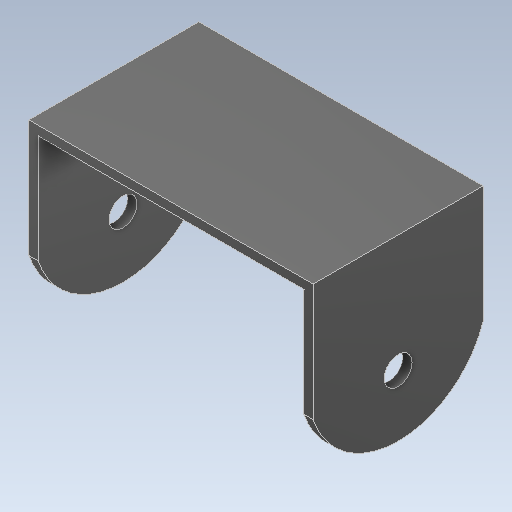
# Autodesk Inventor part: atassolar
Saved by Autodesk Inventor 2025.1 (Build 291241000, 241)
## iProperties
Created: 2024-11-08
Part Number: atassolar
Material: Aluminum 6061
Document SubType Name: Modeling
Designer: ramad
Density: 2.7 g/cm^3
Appearance: Aluminum - Flat
Author: ramad
Autodesk Inventor part; units mm, degrees
ref_plane "YZ Plane" through (0, 0, 0) normal (1, 0, 0) x (0, 1, 0)
ref_plane "XZ Plane" through (0, 0, 0) normal (0, 1, 0) x (-1, 0, 0)
ref_plane "XY Plane" through (0, 0, 0) normal (0, 0, 1) x (1, 0, 0)
sketch "Sketch1" plane through (0, 0, 0) normal (0, 1, 0) x (-1, 0, 0)
  line L0 (-43, 27.5) -> (43, 27.5)
  line L1 (43, 27.5) -> (43, -27.5)
  line L2 (43, -27.5) -> (-43, -27.5)
  line L3 (-43, -27.5) -> (-43, 27.5)
  line L4 (-43, 27.5) -> (43, -27.5) construction
  line L5 (43, 27.5) -> (-43, -27.5) construction
  line L6 (43, -27.5) -> (46, -27.5)
  line L7 (46, -27.5) -> (46, 27.5)
  line L8 (46, 27.5) -> (43, 27.5)
  line L9 (43, 27.5) -> (43, -27.5)
  line L10 (-43, -27.5) -> (-46, -27.5)
  line L11 (-46, -27.5) -> (-46, 27.5)
  line L12 (-46, 27.5) -> (-43, 27.5)
  line L13 (-43, 27.5) -> (-43, -27.5)
  point P0 (0, 0)
  dimension "d0" = 86
  dimension "d1" = 55
  dimension "d2" = 3
  dimension "d3" = 55
  dimension "d4" = 3
  constraints: 28 end point, 6 parallel, 3 horizontal, 3 perpendicular, 2 midpoint, 1 point on line
  measures "d0" distance of L1.end L2.end
  measures "d1" distance of L0.end L1.end
  measures "d2" distance of L8.end L7.end
  measures "d3" distance of L7.end L6.end
  measures "d4" distance of L11.end L12.end
extrude "Extrusion1" add sketch "Sketch1" along normal blind 3 contours L0 L1 L2 L3
extrude "Extrusion2" add sketch "Sketch1" along normal blind 3 contours L3 L10 L11 L12 | L8 L7 L6 L1
extrude "Extrusion3" add sketch "Sketch1" against normal blind 35 contours L3 L10 L11 L12 | L8 L7 L6 L1
sketch "Sketch2" plane through (46, 3, 27.5) normal (1, 0, 0) x (0, 0, -1)
  line L0 (0, -3) -> (0, -38) projected
  line L1 (0, -38) -> (55, -38) projected
  arc A0 (0, -38) -> (55, -38) centre (27.5, -28.794) ccw
  point P0 (27.5, -3)
  dimension "d11" = 29
  constraints: 2 point on circle, 1 centre point
  measures "d11" radius of A0
extrude "Extrusion4" add sketch "Sketch2" against normal up to surface (3 mm away)
mirror "Mirror1" about plane through (0, 0, 0) normal (1, 0, 0) of "Extrusion4"
sketch "Sketch3" plane through (-46, 3, -27.5) normal (-1, 0, 0) x (0, 0, 1)
  circle A0 centre (27.5, -38) radius 4.5
  point P0 (27.5, -3)
  point P1 (0, -38)
  dimension "d14" = 9
  constraints: 1 centre point, 1 horizontal alignment
  measures "d14" diameter of A0
extrude "Extrusion5" cut sketch "Sketch3" against normal blind 106.25
body "Solid1"
